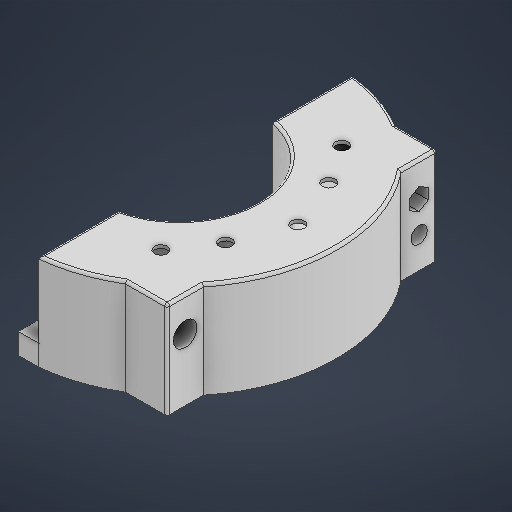
# Autodesk Inventor part: buoy version 16
Saved by Autodesk Inventor 2026 (Build 300175050, 175E)
## iProperties
Created: 2025-06-23
Part Number: buoy version 16
Material: Generic
Document SubType Name: Modeling
Designer: localuser
Density: 1 g/cm^3
Appearance: Default
Author: localuser
Autodesk Inventor part; units mm, degrees
ref_plane "YZ Plane" through (0, 0, 0) normal (1, 0, 0) x (0, 1, 0)
ref_plane "XZ Plane" through (0, 0, 0) normal (0, 1, 0) x (-1, 0, 0)
ref_plane "XY Plane" through (0, 0, 0) normal (0, 0, 1) x (1, 0, 0)
sketch "Sketch1" plane through (0, 0, 0) normal (0, 1, 0) x (-1, 0, 0)
  circle A0 centre (0, 0) radius 30.5
  circle A1 centre (0, 0) radius 61
  line L0 (0, 0) -> (0, 30.5)
  line L1 (0, 30.5) -> (0, -30.5)
  line L2 (0, 30.5) -> (6.35, 30.5)
  line L3 (6.35, 30.5) -> (-6.35, 30.5)
  line L4 (0, -30.5) -> (6.35, -30.5)
  line L5 (6.35, -30.5) -> (-6.35, -30.5)
  line L6 (6.35, 30.5) -> (6.35, 29.8317)
  line L7 (-6.35, 30.5) -> (-6.35, 29.8317)
  line L8 (-6.35, -30.5) -> (-6.35, -29.8317)
  line L9 (6.35, -30.5) -> (6.35, -29.8317)
  line L10 (-6.35, 29.8317) -> (-6.35, 60.6686)
  line L11 (6.35, 29.8317) -> (6.35, 60.6686)
  line L12 (6.35, -29.8317) -> (6.35, -60.6686)
  line L13 (-6.35, -29.8317) -> (-6.35, -60.6686)
  line L14 (-6.35, 60.6686) -> (-6.35, 45.2501)
  line L15 (-6.35, -60.6686) -> (-6.35, -45.2501)
  line L16 (-6.35, 45.2501) -> (-6.35, 38.2501)
  line L17 (-6.35, 38.2501) -> (-6.35, 52.2501)
  line L18 (-6.35, -45.2501) -> (-6.35, -38.2501)
  line L19 (-6.35, -38.2501) -> (-6.35, -52.2501)
  line L20 (-6.35, 38.2501) -> (-47.5177, 38.2501)
  line L21 (-6.35, -38.2501) -> (-47.5177, -38.2501)
  line L22 (-47.5177, 38.2501) -> (-47.5177, 52.2501)
  line L23 (-47.5177, 52.2501) -> (-6.35, 52.2501)
  line L24 (-47.5177, -38.2501) -> (-47.5177, -52.2501)
  line L25 (-47.5177, -52.2501) -> (-6.35, -52.2501)
  point P0 (-31.479, -52.2501)
  point P1 (-31.479, 52.2501)
  dimension "d0" = 61
  dimension "d1" = 122
  dimension "d3" = 6.35
  dimension "d4" = 12.7
  dimension "d5" = 6.35
  dimension "d6" = 12.7
  dimension "d7" = 7
  dimension "d8" = 14
  dimension "d9" = 7
  dimension "d10" = 14
  dimension "d11" = 14
  dimension "d12" = 14
  constraints: 52 end point, 13 point on line, 12 point on circle, 3 vertical, 2 centre point, 2 coincident, 2 horizontal, 2 midpoint, 2 parallel, 2 perpendicular, 1 tangent
  measures "d0" diameter of A0
  measures "d1" diameter of A1
  measures "d3" distance of L0.end L2.end
  measures "d4" distance of L2.end L3.end
  measures "d5" distance of L1.end L4.end
  measures "d6" distance of L4.end L5.end
  measures "d7" distance of L14.end L16.end
  measures "d8" distance of L16.end L17.end
  measures "d9" distance of L15.end L18.end
  measures "d10" distance of L18.end L19.end
  measures "d11" distance of L20.end L22.end
  measures "d12" distance of L21.end L24.end
extrude "Extrusion1" add sketch "Sketch1" along normal blind 36 contours A0 L8 L13 L21 A1 L20 L10 L7 | L20 A1 L23 L10 | L10 L23 A1 | L13 L25 A1 L21 | A1 L25 L13 | L22 L23 A1 | A1 L25 L24
sketch "Sketch2" plane through (47.5177, 0, 52.2501) normal (1, 0, 0) x (0, 0, -1)
  line L0 (0, 0) -> (0, 36) projected
  line L1 (0, 36) -> (7, 36)
  line L2 (22.4185, 36) -> (-8.4185, 36) projected
  line L3 (7, 36) -> (7, 24)
  line L4 (22.4185, 0) -> (-8.4185, 0) projected
  line L5 (7, 24) -> (7, 12)
  line L6 (112.9187, 36) -> (82.0818, 36) projected
  line L7 (97.5002, 36) -> (97.5002, 24)
  line L8 (97.5002, 24) -> (97.5002, 12)
  circle A0 centre (97.5002, 24) radius 4.2
  line L9 (97.5002, 28.2) -> (101.1375, 26.1)
  line L10 (101.1375, 26.1) -> (101.1375, 21.9)
  line L11 (101.1375, 21.9) -> (97.5002, 19.8)
  line L12 (97.5002, 19.8) -> (93.8629, 21.9)
  line L13 (93.8629, 21.9) -> (93.8629, 26.1)
  line L14 (93.8629, 26.1) -> (97.5002, 28.2)
  circle A1 centre (7, 24) radius 4.572
  point P0 (52.2501, 0)
  dimension "d19" = 8.4
  dimension "d15" = 12
  dimension "d16" = 12
  dimension "d17" = 12
  dimension "d18" = 12
  dimension "d20" = 9.144
  constraints: 22 end point, 3 coincident, 2 midpoint, 2 point on line, 1 centre point, 1 perpendicular, 1 vertical, 1 vertical alignment, 15 other
  measures "d15" distance of L1.end L3.end
  measures "d16" distance of L3.end L5.end
  measures "d17" distance of L7.start L7.end
  measures "d18" distance of L7.end L8.end
  measures "d20" diameter of A1
extrude "Extrusion2" cut sketch "Sketch2" against normal blind 19.05 contours A1 L5 L3 | L3 L5 A1 | L9 L10 L11 L8 L7 | L7 L8 L12 L13 L14
sketch "Sketch4" plane through (28.4677, 0, 52.2501) normal (1, 0, 0) x (0, 0, -1)
  line L0 (97.5002, 28.2) -> (101.1375, 26.1) projected
  line L1 (97.5002, 28.2) -> (97.5002, 19.8)
  line L2 (97.5002, 19.8) -> (97.5002, 24)
  circle A0 centre (7, 24) radius 4.572 projected
  line L3 (6.3611, 28.2) -> (7, 24)
  line L4 (7, 24) -> (4.1588, 20.418)
  line L5 (7, 24) -> (11.0612, 21.9)
  point P0 (52.2501, 0)
  constraints: 10 end point, 2 point on circle, 1 midpoint, 1 vertical
hole "Hole1" at (28.4677, 24, 45.2501) at (28.4677, 24, -45.2501) direction (-1, 0, 0) diameter 4.064 depth 25.4 tip angle 118
sketch "Sketch5" plane through (47.5177, 0, -38.2501) normal (1, 0, 0) x (0, 0, -1)
  line L0 (0, 0) -> (14, 0) projected
  line L1 (7, 0) -> (7, 12)
  point P0 (-38.2501, 0)
  dimension "d30" = 12
  constraints: 2 end point, 1 midpoint, 1 vertical
  measures "d30" distance of L1.start L1.end
hole "Hole2" at (47.5177, 12, -45.2501) direction (-1, 0, 0) diameter 6.35 depth 42 tip angle 118
sketch "Sketch6" plane through (6.35, 0, -60.6686) normal (-1, 0, 0) x (0, 0, 1)
  circle A0 centre (15.4185, 12) radius 3.175 projected
  circle A1 centre (15.4185, 12) radius 5.6
  line L0 (15.4185, 6.4) -> (10.5687, 9.2)
  line L1 (10.5687, 9.2) -> (10.5687, 14.8)
  line L2 (10.5687, 14.8) -> (15.4185, 17.6)
  line L3 (15.4185, 17.6) -> (20.2682, 14.8)
  line L4 (20.2682, 14.8) -> (20.2682, 9.2)
  line L5 (20.2682, 9.2) -> (15.4185, 6.4)
  point P0 (60.6686, 0)
  dimension "d38" = 11.2
  constraints: 12 end point, 2 coincident, 1 vertical alignment, 15 other
extrude "Extrusion3" cut sketch "Sketch6" against normal blind 25 contours L4 L5 L0 L1 L2 L3
sketch "Sketch7" plane through (6.35, 0, -60.6686) normal (-1, 0, 0) x (0, 0, 1)
  line L0 (0, 0) -> (0, 36) projected
  line L1 (0, 0) -> (30.8369, 0) projected
  line L2 (0, 0) -> (8, 0)
  line L3 (8, 0) -> (8, 8)
  line L4 (8, 8) -> (0, 8)
  line L5 (0, 8) -> (0, 0)
  line L6 (121.3372, 0) -> (112.9187, 0) projected
  line L7 (121.3372, 0) -> (113.3372, 0)
  line L8 (113.3372, 0) -> (113.3372, 8)
  line L9 (113.3372, 8) -> (121.3372, 8)
  line L10 (121.3372, 8) -> (121.3372, 0)
  point P0 (60.6686, 0)
  dimension "d42" = 8
  dimension "d43" = 8
  dimension "d44" = 8
  dimension "d45" = 8
  constraints: 16 end point, 5 perpendicular, 3 point on line, 1 collinear
  measures "d42" distance of L0.start L2.end
  measures "d43" distance of L2.end L3.end
  measures "d44" distance of L6.start L7.end
  measures "d45" distance of L7.end L8.end
extrude "Extrusion4" add sketch "Sketch7" along normal blind 8
shell "Shell1" thickness 1.25 removed faces 1 at (32.9179, 36, 37.912)
sketch "Sketch8" plane through (0, 36, 0) normal (0, 1, 0) x (1, 0, 0)
  arc A0 (6.35, -29.8317) -> (6.35, 29.8317) centre (0, 0) ccw projected
  arc A1 (6.35, -29.8317) -> (6.35, 29.7752) centre (-0.006, -0.0282) ccw
  line L0 (47.5177, 52.2501) -> (31.479, 52.2501) projected
  line L1 (6.35, 60.6686) -> (6.35, 29.8317) projected
  arc A2 (31.479, 52.2501) -> (6.35, 60.6686) centre (0, 0) ccw
  line L2 (47.5177, -52.2501) -> (47.5177, -38.2501) projected
  arc A3 (47.5177, -38.2501) -> (47.5177, 38.2501) centre (0, 0) ccw
  circle A4 centre (0, 0) radius 30.5
  circle A5 centre (0, 0) radius 61
  line L3 (31.479, 52.2501) -> (47.5177, 52.2501)
  line L4 (47.5177, -38.2501) -> (47.5177, -52.2501)
  line L5 (31.479, -52.2501) -> (47.5177, -52.2501) projected
  line L6 (47.5177, -52.2501) -> (31.479, -52.2501)
  line L7 (6.35, -29.8317) -> (6.35, -52.6686) projected
  line L8 (6.35, -29.8317) -> (6.35, -60.6686)
  line L9 (6.35, 29.7752) -> (6.35, 60.6686)
  arc A6 (6.35, -60.6686) -> (31.479, -52.2501) centre (0, 0) ccw
  point P0 (47.5177, 38.2501)
  dimension "d49" = 61
  dimension "d50" = 122
  constraints: 10 end point, 9 point on circle, 6 centre point, 4 collinear, 2 coincident, 1 concentric
  measures "d49" diameter of A4
  measures "d50" diameter of A5
extrude "Extrusion5" add sketch "Sketch8" along normal blind 1.25 contours A0 L1 A2 A5 A3 L8 L7 | A5 L2 L5
sketch "Sketch9" plane through (0, 36, 0) normal (0, 1, 0) x (1, 0, 0)
  line L0 (47.5177, 38.2501) -> (47.5177, 52.2501) projected
  line L1 (47.5177, 52.2501) -> (31.479, 52.2501) projected
  line L2 (47.5177, 52.2501) -> (31.479, 52.2501)
  line L3 (31.479, 52.2501) -> (47.5177, 52.2501)
  line L4 (47.5177, 38.2501) -> (47.5177, 52.2501)
  arc A0 (47.5177, 38.2501) -> (31.479, 52.2501) centre (0, 0) ccw
  point P0 (0, 0)
  constraints: 6 end point, 3 collinear, 2 point on circle, 1 centre point
extrude "Extrusion6" add sketch "Sketch9" along normal blind 1.25
fillet "Fillet1" radius 1 12 edges at (39.4983, 37.25, -52.2501) (47.5177, 37.25, -45.2501) (61, 37.25, 0) (19.3772, 37.25, -57.8405) (47.5177, 37.25, 45.2501) (39.4983, 37.25, 52.2501) (19.3772, 37.25, 57.8405) (30.5, 37.25, 0) (6.35, 37.25, -45.2501) (6.35, 37.25, 45.2501) (47.5177, 18.625, -52.2501) (47.5177, 18.625, 52.2501)
sketch "Sketch10" plane through (0, 37.25, 0) normal (0, 1, 0) x (1, 0, 0)
  arc A0 (7.6, -30.827) -> (7.6, 30.827) centre (0, 0) ccw projected
  line L0 (31.75, 0) -> (60, 0)
  arc A1 (46.5177, -37.896) -> (46.5177, 37.896) centre (0, 0) ccw projected
  line L1 (45.875, 0) -> (45.875, -20)
  line L2 (45.875, -20) -> (37.875, -20)
  line L3 (37.875, -20) -> (37.875, 20)
  line L4 (37.875, 20) -> (37.875, 35)
  line L5 (37.875, 35) -> (27.875, 35)
  line L6 (27.875, 35) -> (27.875, -35)
  dimension "d56" = 20
  dimension "d57" = 8
  dimension "d58" = 40
  dimension "d59" = 15
  dimension "d60" = 10
  dimension "d61" = 70
  constraints: 14 end point, 4 perpendicular, 2 point on circle, 1 horizontal, 1 midpoint, 1 point on line, 1 vertical
  measures "d56" distance of L1.start L1.end
  measures "d57" distance of L1.end L2.end
  measures "d58" distance of L2.end L3.end
  measures "d59" distance of L3.end L4.end
  measures "d60" distance of L4.end L5.end
  measures "d61" distance of L5.end L6.end
hole "Hole3" at (27.875, 37.25, 35) at (27.875, 37.25, -35) at (37.875, 37.25, 20) at (37.875, 37.25, -20) at (45.875, 37.25, 0) direction (0, -1, 0) diameter 5 depth 2 tip angle 118
body "Solid1"
